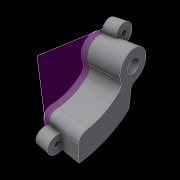
# Autodesk Inventor part: Brake Pad
Saved by Autodesk Inventor 2016 (Build 200138000, 138)
## iProperties
Created: 2012-08-08
Part Number: Brake Pad
Material: Generic
Document SubType Name: Modeling
Designer: John
Density: 1 g/cm^3
Appearance: Default
Author: John
Autodesk Inventor part; units mm, degrees
ref_plane "YZ Plane" through (0, 0, 0) normal (1, 0, 0) x (0, 1, 0)
ref_plane "XZ Plane" through (0, 0, 0) normal (0, 1, 0) x (-1, 0, 0)
ref_plane "XY Plane" through (0, 0, 0) normal (0, 0, 1) x (1, 0, 0)
sketch "Sketch1" plane through (0, 0, 0) normal (1, 0, 0) x (0, 1, 0)
  arc A0 (-0.635, -11.743) -> (7.62, -8.9576) centre (0, 0) ccw
  arc A1 (-0.635, -7.5935) -> (6.0473, -4.6363) centre (0, 0) ccw
  circle A2 centre (7.62, -3.048) radius 2.2352
  line L0 (7.62, -5.2832) -> (7.62, -8.9576)
  line L1 (-0.635, -11.743) -> (-0.635, -7.5935)
  dimension "d0" = 11.7602
  dimension "d1" = 7.62
  dimension "d8" = 2.2352
  dimension "d9" = 7.62
  dimension "d10" = 3.048
  dimension "d11" = 0.635
  constraints: 6 point on circle, 4 end point, 3 centre point, 2 coincident, 1 parallel, 1 vertical, 1 vertical alignment
  measures "d0" radius of A0
  measures "d1" radius of A1
  measures "d8" radius of A2
  measures "d9" horizontal distance of A2.centre A1.centre
  measures "d10" vertical distance of A0.centre A2.centre
  measures "d11" distance from line of point (0, 0) L1
extrude "Extrusion1" add sketch "Sketch1" along normal blind 5.7912
fillet "Fillet1" radius 1.27 1 edges at (2.8956, 6.0473, -4.6363)
fillet "Fillet2" radius 0.889 1 edges at (2.8956, 7.62, -5.2832)
fillet "Fillet3" radius 0.889 1 edges at (2.8956, 7.62, -8.9576)
ref_plane "Work Plane1" through (1.016, 0, 0) normal (-1, 0, 0) x (0, 0, 1)
sketch "Sketch2" plane through (1.016, 0, 0) normal (-1, 0, 0) x (0, 0, 1)
  arc A0 (-3.9958, 5.5957) -> (-5.4412, 5.3346) centre (-4.5343, 4.4455) ccw projected
  arc A1 (-5.4412, 5.3346) -> (-7.5935, -0.635) centre (0, 0) ccw projected
  line L0 (-7.5935, -0.635) -> (-11.743, -0.635) projected
  arc A2 (-9.2349, 7.2814) -> (-11.743, -0.635) centre (0, 0) ccw projected
  arc A3 (-8.5368, 7.62) -> (-9.2349, 7.2814) centre (-8.5368, 6.731) ccw projected
  line L1 (-8.5368, 7.62) -> (-6.043, 7.62) projected
  arc A4 (-6.043, 7.62) -> (-5.1908, 8.256) centre (-6.043, 8.509) ccw projected
  arc A5 (-3.9958, 5.5957) -> (-5.1908, 8.256) centre (-3.048, 7.62) ccw projected
  circle A6 centre (-10.414, -1.27) radius 1.397
  circle A7 centre (-0.635, 9.144) radius 1.397
  dimension "d18" = 1.397
  dimension "d19" = 1.27
  dimension "d20" = 10.414
  dimension "d21" = 1.397
  dimension "d22" = 0.635
  dimension "d23" = 9.144
  constraints: 2 centre point
  measures "d18" radius of A6
  measures "d19" vertical distance of point (0, 0) A6.centre
  measures "d20" horizontal distance of point (0, 0) A6.centre
  measures "d21" radius of A7
  measures "d22" horizontal distance of point (0, 0) A7.centre
  measures "d23" vertical distance of point (0, 0) A7.centre
extrude "Extrusion2" add sketch "Sketch2" against normal blind 2.032 contours A7 A5 | A5 A7 | A6 L0 | L0 A6
fillet "Fillet4" radius 1.27 1 edges at (2.8956, -0.635, -7.5935)
sketch "Sketch3" plane through (3.048, 0, 0) normal (1, 0, 0) x (0, 0, -1)
  arc A0 (1.9639, 9.5747) -> (0.8171, 7.7589) centre (0.635, 9.144) ccw projected
  line L0 (9.1697, -0.635) -> (11.6583, -0.635) projected
  arc A1 (9.1697, -0.635) -> (11.6583, -0.635) centre (10.414, -1.27) ccw projected
  point P0 (0, 0)
hole "Hole1" at (3.048, -1.27, -10.414) at (3.048, 9.144, -0.635) direction (-1, 0, 0) diameter 1.016 end through all
sketch "Sketch4" plane through (5.7912, 0, 0) normal (1, 0, 0) x (0, 0, -1)
  arc A0 (5.1908, 8.256) -> (3.9958, 5.5957) centre (3.048, 7.62) ccw projected
hole "Hole2" at (5.7912, 7.62, -3.048) direction (-1, 0, 0) diameter 2.032 end through all
body "Solid1"
